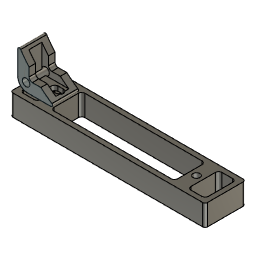
Pi Cluser Fan Spacer and corner v2 (Autodesk Fusion 360 design; units mm, degrees)
Autodesk Fusion 360 part; units mm, degrees
mesh "Mesh1" [no effect]
sketch "Sketch1" plane through (0, 0, 0) normal (0, 0, 1) x (1, 0, 0)
  line L0 (1.5, 0) -> (118.5, 0)
  line L1 (120, 1.5) -> (120, 23.5)
  line L2 (118.5, 25) -> (1.5, 25)
  line L3 (0, 23.5) -> (0, 1.5)
  arc A0 (1.5, 25) -> (0, 23.5) centre (1.5, 23.5) ccw
  arc A1 (0, 1.5) -> (1.5, 0) centre (1.5, 1.5) ccw
  arc A2 (120, 23.5) -> (118.5, 25) centre (118.5, 23.5) ccw
  arc A3 (118.5, 0) -> (120, 1.5) centre (118.5, 1.5) ccw
  line L4 (3, 20) -> (3, 5)
  line L5 (117, 5) -> (117, 20)
  line L6 (21.8786, 20) -> (21.8786, 5)
  line L7 (13.6399, 5) -> (13.6399, 20)
  line L8 (98.1214, 20) -> (98.1214, 5)
  line L9 (106.3601, 5) -> (106.3601, 20)
  circle A4 centre (17.7755, 12.4934) radius 2.1383
  circle A5 centre (102.2245, 12.4934) radius 2.1383
  line L10 (115, 22) -> (108.3601, 22)
  line L11 (108.3601, 3) -> (115, 3)
  arc A6 (108.3601, 22) -> (106.3601, 20) centre (108.3601, 20) ccw
  arc A7 (117, 20) -> (115, 22) centre (115, 20) ccw
  arc A8 (115, 3) -> (117, 5) centre (115, 5) ccw
  arc A9 (106.3601, 5) -> (108.3601, 3) centre (108.3601, 5) ccw
  arc A10 (96.1214, 3) -> (98.1214, 5) centre (96.1214, 5) ccw
  arc A11 (98.1214, 20) -> (96.1214, 22) centre (96.1214, 20) ccw
  line L12 (96.1214, 22) -> (23.8786, 22)
  line L13 (11.6399, 22) -> (5, 22)
  line L14 (5, 3) -> (11.6399, 3)
  line L15 (23.8786, 3) -> (96.1214, 3)
  arc A12 (23.8786, 22) -> (21.8786, 20) centre (23.8786, 20) ccw
  arc A13 (13.6399, 20) -> (11.6399, 22) centre (11.6399, 20) ccw
  arc A14 (5, 22) -> (3, 20) centre (5, 20) ccw
  arc A15 (3, 5) -> (5, 3) centre (5, 5) ccw
  arc A16 (11.6399, 3) -> (13.6399, 5) centre (11.6399, 5) ccw
  arc A17 (21.8786, 5) -> (23.8786, 3) centre (23.8786, 5) ccw
  dimension "d1" = 1.5
  dimension "d3" = 2
  dimension "d4" = 2
  dimension "d5" = 2
  dimension "d6" = 2
  constraint horizontal L0
  constraint vertical L1
  constraint horizontal L2
  constraint vertical L3
  constraint tangent L2 A0
  constraint tangent L3 A0
  constraint tangent L0 A1
  constraint tangent L3 A1
  constraint equal A0 A1
  constraint tangent L1 A2
  constraint tangent L2 A2
  constraint equal A0 A2
  constraint tangent L0 A3
  constraint tangent L1 A3
  constraint equal A0 A3
  constraint vertical L6
  constraint vertical L7
  constraint parallel L3 L4
  constraint parallel L0 L14
  constraint parallel L1 L5
  constraint parallel L2 L10
  constraint collinear L10 L12
  constraint collinear L11 L14
  constraint tangent L10 A6
  constraint tangent L9 A6
  constraint tangent L10 A7
  constraint tangent L5 A7
  constraint equal A6 A7
  constraint tangent L5 A8
  constraint tangent L11 A8
  constraint equal A6 A8
  constraint tangent L11 A9
  constraint tangent L9 A9
  constraint equal A6 A9
  constraint tangent L8 A10
  constraint tangent A10 L14
  constraint equal A6 A10
  constraint tangent L8 A11
  constraint tangent A11 L12
  constraint equal A6 A11
  constraint collinear L12 L13
  constraint collinear L14 L15
  constraint tangent L12 A12
  constraint tangent L6 A12
  constraint tangent L7 A13
  constraint tangent L13 A13
  constraint equal A12 A13
  constraint tangent L13 A14
  constraint tangent L4 A14
  constraint equal A12 A14
  constraint tangent L4 A15
  constraint tangent L14 A15
  constraint equal A12 A15
  constraint tangent L14 A16
  constraint tangent L7 A16
  constraint tangent L6 A17
  constraint tangent L15 A17
  measures "d1" radius of A0
  measures "d3" radius of A6
  measures "d4" radius of A12
  measures "d5" radius of A16
  measures "d6" radius of A17
extrude "Extrude1" add sketch "Sketch1" along normal blind 13 makes body 1
sketch "Sketch2" plane through (0, 0, 0) normal (0, 1, 0) x (1, 0, 0)
  line L0 (0, -13) -> (0, -37)
  line L1 (0, -13) -> (24, -13)
  line L2 (7.5, -17) -> (112.5, -17)
  line L3 (120, -13) -> (120, -133)
  line L4 (120, -73) -> (60, -73)
  arc A0 (120, -109.0555) -> (102, -17) centre (60, -73) ccw
  line L5 (60, -73) -> (60, -20.5)
  line L6 (-600, 200) -> (-480, 200)
  line L7 (-480, 200) -> (-480, 80)
  line L8 (-480, 80) -> (-600, 80)
  line L9 (-600, 80) -> (-600, 200)
  line L10 (-592.5, 192.5) -> (-487.5, 192.5)
  line L11 (-487.5, 192.5) -> (-487.5, 87.5)
  line L12 (-487.5, 87.5) -> (-592.5, 87.5)
  line L13 (-592.5, 87.5) -> (-592.5, 192.5)
  circle A1 centre (-592.5, 192.5) radius 2.25
  line L14 (0, -13) -> (0, -133)
  line L15 (0, -133) -> (120, -133)
  line L16 (120, -133) -> (120, -13)
  line L17 (6.7, -126.3) -> (113.3, -126.3)
  line L18 (113.3, -126.3) -> (113.3, -19.7)
  line L19 (5.2, -18.2) -> (24, -18.2) construction
  line L20 (5.2, -18.2) -> (5.2, -37) construction
  circle A2 centre (5.2, -18.2) radius 2.3
  line L21 (7, -22) -> (7, -27.2725)
  line L22 (9, -20) -> (14.2725, -20)
  arc A3 (9, -20) -> (7, -22) centre (9, -22) ccw
  arc A4 (7, -27.2725) -> (0, -36.9445) centre (60, -73) ccw
  arc A5 (0, -109.0555) -> (102, -17) centre (60, -73) ccw
  arc A6 (23.9445, -13) -> (14.2725, -20) centre (60, -73) ccw
  point P0 (60, -20)
  point P1 (120, -73)
  dimension "d9" = 24
  dimension "d10" = 24
  dimension "d11" = 105
  dimension "d14" = 120
  dimension "d15" = 60
  dimension "d16" = 140
  dimension "d18" = 52.5
  dimension "d19" = 120
  dimension "d20" = 120
  dimension "d21" = 7.5
  dimension "d22" = 4.5
  dimension "d23" = 120
  dimension "d24" = 120
  dimension "d27" = 5.2
  dimension "d28" = 4.6
  dimension "d30" = 2
  dimension "d31" = 140
  constraint vertical L0
  constraint perpendicular L0 L1
  constraint horizontal L2
  constraint perpendicular L2 L3
  constraint midpoint L3 P1
  constraint coincident P1 L4.start
  constraint perpendicular L3 L4
  constraint coincident L4.end A0.centre
  constraint coincident L3 A0.start
  constraint coincident L2 A0.end
  constraint perpendicular L4 L5
  constraint horizontal L6
  constraint vertical L7
  constraint horizontal L8
  constraint vertical L9
  constraint coincident L10.start L13.end
  constraint vertical L14
  constraint horizontal L15
  constraint vertical L16
  constraint coincident L19.start L20.start
  constraint parallel L15 L17
  constraint parallel L16 L18
  constraint parallel L0 L21
  constraint parallel L1 L22
  constraint tangent L21 A3
  constraint tangent L22 A3
  constraint coincident L0 A4.end
  constraint coincident L14 A5.start
  constraint concentric A4 A5
  constraint coincident L1 A6.start
  constraint concentric A5 A6
  measures "d9" distance of L0.start L0.end
  measures "d10" distance of L0.start L1.end
  measures "d11" distance of L2.start L2.end
  measures "d14" distance of L3.start L3.end
  measures "d15" distance of P1 L4.end
  measures "d16" diameter of A0
  measures "d18" distance of L4.end L5.end
  measures "d19" distance of L6.start L6.end
  measures "d20" distance of L6.start L8.end
  measures "d22" diameter of A1
  measures "d23" distance of L3.start L0.start
  measures "d24" distance of L3.start L3.end
  measures "d28" diameter of A2
  measures "d30" radius of A3
  measures "d31" diameter of A5
extrude "Extrude1'" add sketch "Sketch2" along normal blind 16 separate body contours L0 L1 L14 L21 L22 A3 A4 A6 makes body 2 in component "Component"
fillet "Fillet1" radius 6 1 edges at (0, 8, 13) on bodies 2 in component "Component"
fillet "Fillet1" radius 1 2 edges at (23.9445, 8, 13) (0, 8, 36.9445) on bodies 2 in component "Component"
sketch "Sketch1 (2)" plane through (0, 0, 0) normal (0, -1, 0) x (1, 0, 0) in component "Component"
  arc A0 (1.831, 34.0595) -> (0, 33.5032) centre (1, 33.5032) ccw
  line L0 (0, 33.5032) -> (0, 19)
  arc A1 (0, 19) -> (6, 13) centre (6, 19) ccw
  line L1 (6, 13) -> (20.5032, 13)
  arc A2 (20.5032, 13) -> (21.0595, 14.831) centre (20.5032, 14) ccw
  arc A3 (14.2725, 20) -> (21.0595, 14.831) centre (60, 73) ccw
  line L2 (14.2725, 20) -> (9, 20)
  arc A4 (7, 22) -> (9, 20) centre (9, 22) ccw
  line L3 (7, 22) -> (7, 27.2725)
  arc A5 (1.831, 34.0595) -> (7, 27.2725) centre (60, 73) ccw
  circle A6 centre (5.2, 18.2) radius 2.3
sketch "Sketch2 (2)" plane through (0, 0, 0) normal (0, -1, 0) x (1, 0, 0) in component "Component"
  line L0 (5.2, 15.9) -> (21, 15.9)
  circle A0 centre (5.2, 18.2) radius 2.3
  line L1 (2.9, 18.2) -> (2.9, 33.7067)
  arc A1 (2.9, 18.2) -> (5.2, 15.9) centre (5.2, 18.2) ccw
  line L2 (2.9, 33.7067) -> (21, 15.9)
  dimension "d36" = 2.3
  constraint horizontal L0
  constraint tangent L0 A0
  constraint perpendicular L0 L1
  constraint tangent A0 L1
  constraint tangent L1 A1
  constraint tangent L0 A1
  measures "d36" radius of A1
extrude "Extrude2" cut sketch "Sketch2 (2)" along normal blind -12 and the other way blind 4 contours L0 A0 L1 L2 bodies 2 in component "Component"
sketch "Sketch3" plane through (0, 0, 13) normal (0, 0, -1) x (1, 0, 0) in component "Component"
  line L0 (20.5032, -16) -> (20.5032, 0)
  line L1 (20.5032, 0) -> (6, 0)
  line L2 (6, 0) -> (6, -16)
  line L3 (6, -16) -> (20.5032, -16)
  line L4 (14.5447, -5.7552) -> (17.7672, -5.7434)
  line L5 (14.5447, -10.2315) -> (17.7672, -10.2433)
  arc A0 (14.5447, -5.7552) -> (14.9898, -10.2331) centre (14.7755, -7.9934) ccw
  arc A1 (16.3572, -6.3931) -> (16.2755, -6.3163) centre (14.7755, -7.9934) ccw
  arc A2 (17.7672, -10.2433) -> (17.7672, -5.7434) centre (17.7755, -7.9934) ccw
  dimension "d41" = 4.5
  dimension "d42" = 4.5
  constraint tangent L4 A2
  constraint coincident L5.start A0
  constraint tangent L5 A2
  constraint concentric A0 A1
  constraint coincident L5 A0.end
  measures "d41" diameter of A2
  measures "d42" diameter of A0
extrude "Extrude3" cut sketch "Sketch3" against normal blind 4 contours L4 L5 A0 A2 bodies 2 in component "Component"
component "Component" placed x (1, 0, 0) y (0, 1, 0) z (0, 0, 1) at (0, 4.5, 0)
